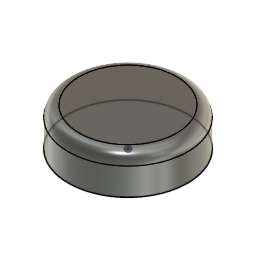
TAPA_TERMO (Autodesk Fusion 360 design; units mm, degrees)
Autodesk Fusion 360 part; units mm, degrees
sketch "Boceto1" plane through (0, 0, 0) normal (0, 0, 1) x (1, 0, 0)
  circle A0 centre (0, 0) radius 55
  dimension "d1" = 110
  constraint coincident A0.centre origin
  measures "d1" diameter of A0
extrude "Extruir1" add sketch "Boceto1" along normal blind 35
hole "Agujero3" at (0, 0, 0) direction (0, 0, 1) diameter 100 depth 25 tip angle 180
thread "Rosca2" "ISO Metric profile 100.0 M100x6 M100x6 6H" major diameter 100.633 minor diameter 93.905 pitch 6 angle 60 resizes the face on face at (4.9784, 49.7515, 16.6667) from (0, 0, 0) to (0, 0, 20)
thread "Rosca3" "ISO Metric profile 100.0 M100x6 M100x6 6H" major diameter 100.633 minor diameter 93.905 pitch 6 angle 60 modelled right hand crest width 1.6155 on face at (4.675, 46.7192, 16.6667) crest through (-46.9525, 0, 1.5)
fillet "Empalme1" radius 10 1 edges at (-51.278, -19.8888, 35)
